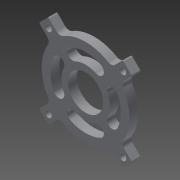
# Autodesk Inventor part: Colossus_7kW_Stator
Saved by Autodesk Inventor 2016 (Build 200138000, 138)
## iProperties
Created: 2014-11-23
Part Number: Colossus_7kW_Stator
Material: Générique
Document SubType Name: Modeling
Designer: Yann
Density: 1 g/cm^3
Appearance: Par défaut
Author: Yann
Autodesk Inventor part; units mm, degrees
ref_plane "YZ Plane" through (0, 0, 0) normal (1, 0, 0) x (0, 1, 0)
ref_plane "XZ Plane" through (0, 0, 0) normal (0, 1, 0) x (-1, 0, 0)
ref_plane "XY Plane" through (0, 0, 0) normal (0, 0, 1) x (1, 0, 0)
sketch "Esquisse1" plane through (0, 0, 0) normal (0, 1, 0) x (-1, 0, 0)
  circle A0 centre (33.9411, 33.9411) radius 3
  line L0 (0, -58.8171) -> (0, 58.8171) projected
  line L1 (-58.8171, 0) -> (58.8171, 0) projected
  line L2 (0, 0) -> (33.9411, 33.9411) construction
  line L3 (26.6119, 35.0971) -> (33.234, 41.7193)
  line L4 (34.6482, 41.7193) -> (41.7193, 34.6482)
  line L5 (41.7193, 33.234) -> (35.0971, 26.6119)
  arc A1 (34.6482, 41.7193) -> (33.234, 41.7193) centre (33.9411, 41.0122) ccw
  arc A2 (41.7193, 33.234) -> (41.7193, 34.6482) centre (41.0122, 33.9411) ccw
  arc A3 (11.636, 24.364) -> (-11.636, 24.364) centre (0, 0) ccw construction
  arc A4 (13.7909, 28.8758) -> (-13.7909, 28.8758) centre (0, 0) ccw
  arc A5 (9.4812, 19.8521) -> (-9.4812, 19.8521) centre (0, 0) ccw
  arc A6 (9.4812, 19.8521) -> (13.7909, 28.8758) centre (11.636, 24.364) ccw
  arc A7 (-13.7909, 28.8758) -> (-9.4812, 19.8521) centre (-11.636, 24.364) ccw
  circle A8 centre (0, 0) radius 16
  arc A9 (20.5123, 34.3402) -> (0, 40) centre (0, 0) ccw
  arc A10 (40, 0) -> (34.3402, 20.5123) centre (0, 0) ccw
  arc A11 (20.5123, 34.3402) -> (26.6119, 35.0971) centre (23.0763, 38.6327) ccw
  arc A12 (35.0971, 26.6119) -> (34.3402, 20.5123) centre (38.6327, 23.0763) ccw
  circle A13 centre (-33.9411, 33.9411) radius 3
  line L6 (0, 0) -> (-33.9411, 33.9411) construction
  line L7 (-35.0971, 26.6119) -> (-41.7193, 33.234)
  line L8 (-41.7193, 34.6482) -> (-34.6482, 41.7193)
  line L9 (-33.234, 41.7193) -> (-26.6119, 35.0971)
  arc A14 (-41.7193, 34.6482) -> (-41.7193, 33.234) centre (-41.0122, 33.9411) ccw
  arc A15 (-33.234, 41.7193) -> (-34.6482, 41.7193) centre (-33.9411, 41.0122) ccw
  arc A16 (-24.364, 11.636) -> (-24.364, -11.636) centre (0, 0) ccw construction
  arc A17 (-28.8758, 13.7909) -> (-28.8758, -13.7909) centre (0, 0) ccw
  arc A18 (-19.8521, 9.4812) -> (-19.8521, -9.4812) centre (0, 0) ccw
  arc A19 (-19.8521, 9.4812) -> (-28.8758, 13.7909) centre (-24.364, 11.636) ccw
  arc A20 (-28.8758, -13.7909) -> (-19.8521, -9.4812) centre (-24.364, -11.636) ccw
  arc A21 (-34.3402, 20.5123) -> (-40, 0) centre (0, 0) ccw
  arc A22 (0, 40) -> (-20.5123, 34.3402) centre (0, 0) ccw
  arc A23 (-34.3402, 20.5123) -> (-35.0971, 26.6119) centre (-38.6327, 23.0763) ccw
  arc A24 (-26.6119, 35.0971) -> (-20.5123, 34.3402) centre (-23.0763, 38.6327) ccw
  circle A25 centre (-33.9411, -33.9411) radius 3
  line L10 (0, 0) -> (-33.9411, -33.9411) construction
  line L11 (-26.6119, -35.0971) -> (-33.234, -41.7193)
  line L12 (-34.6482, -41.7193) -> (-41.7193, -34.6482)
  line L13 (-41.7193, -33.234) -> (-35.0971, -26.6119)
  arc A26 (-34.6482, -41.7193) -> (-33.234, -41.7193) centre (-33.9411, -41.0122) ccw
  arc A27 (-41.7193, -33.234) -> (-41.7193, -34.6482) centre (-41.0122, -33.9411) ccw
  arc A28 (-11.636, -24.364) -> (11.636, -24.364) centre (0, 0) ccw construction
  arc A29 (-13.7909, -28.8758) -> (13.7909, -28.8758) centre (0, 0) ccw
  arc A30 (-9.4812, -19.8521) -> (9.4812, -19.8521) centre (0, 0) ccw
  arc A31 (-9.4812, -19.8521) -> (-13.7909, -28.8758) centre (-11.636, -24.364) ccw
  arc A32 (13.7909, -28.8758) -> (9.4812, -19.8521) centre (11.636, -24.364) ccw
  arc A33 (-20.5123, -34.3402) -> (0, -40) centre (0, 0) ccw
  arc A34 (-40, 0) -> (-34.3402, -20.5123) centre (0, 0) ccw
  arc A35 (-20.5123, -34.3402) -> (-26.6119, -35.0971) centre (-23.0763, -38.6327) ccw
  arc A36 (-35.0971, -26.6119) -> (-34.3402, -20.5123) centre (-38.6327, -23.0763) ccw
  circle A37 centre (33.9411, -33.9411) radius 3
  line L14 (0, 0) -> (33.9411, -33.9411) construction
  line L15 (35.0971, -26.6119) -> (41.7193, -33.234)
  line L16 (41.7193, -34.6482) -> (34.6482, -41.7193)
  line L17 (33.234, -41.7193) -> (26.6119, -35.0971)
  arc A38 (41.7193, -34.6482) -> (41.7193, -33.234) centre (41.0122, -33.9411) ccw
  arc A39 (33.234, -41.7193) -> (34.6482, -41.7193) centre (33.9411, -41.0122) ccw
  arc A40 (24.364, -11.636) -> (24.364, 11.636) centre (0, 0) ccw construction
  arc A41 (28.8758, -13.7909) -> (28.8758, 13.7909) centre (0, 0) ccw
  arc A42 (19.8521, -9.4812) -> (19.8521, 9.4812) centre (0, 0) ccw
  arc A43 (19.8521, -9.4812) -> (28.8758, -13.7909) centre (24.364, -11.636) ccw
  arc A44 (28.8758, 13.7909) -> (19.8521, 9.4812) centre (24.364, 11.636) ccw
  arc A45 (34.3402, -20.5123) -> (40, 0) centre (0, 0) ccw
  arc A46 (0, -40) -> (20.5123, -34.3402) centre (0, 0) ccw
  arc A47 (34.3402, -20.5123) -> (35.0971, -26.6119) centre (38.6327, -23.0763) ccw
  arc A48 (26.6119, -35.0971) -> (20.5123, -34.3402) centre (23.0763, -38.6327) ccw
  circle A49 centre (0, 0) radius 16 construction
  point P0 (23.7216, 32.2069)
  point P1 (32.2069, 23.7216)
  point P2 (-32.2069, 23.7216)
  point P3 (-23.7216, 32.2069)
  point P4 (-23.7216, -32.2069)
  point P5 (-32.2069, -23.7216)
  point P6 (32.2069, -23.7216)
  point P7 (23.7216, -32.2069)
  dimension "d1" = 6
  dimension "d2" = 48
  dimension "d3" = 6
  dimension "d4" = 6
  dimension "d5" = 45
  dimension "d6" = 1
  dimension "d9" = 10
  dimension "d10" = 9
  dimension "d11" = 40
  dimension "d12" = 5
  dimension "d13" = 27
  constraints: 96 point on circle, 49 centre point, 32 end point, 17 coincident, 13 tangent, 8 point on line, 3 equal radius, 2 perpendicular, 1 parallel, 1 symmetric about line, 1 other
  measures "d1" diameter of A0
  measures "d2" distance of L2.start L2.end
  measures "d3" distance from line of L4 L2.end
  measures "d4" distance from line of L2.end L3
  measures "d5" angle of L1 L2
  measures "d6" radius of A1
  measures "d9" radial gap between concentric circles of A5 A4
  measures "d10" distance from line of A3.start L2
  measures "d11" radius of A9
  measures "d12" radius of A11
  measures "d13" radius of A3
extrude "Extrusion1" add sketch "Esquisse1" along normal blind 8 contours A33 A35 L11 A26 L12 A27 L13 A36 A34 L1 A17 A20 A18 A8 L0 A30 A31 A29 | L0 A29 A32 A30 A8 L1 A42 A43 A41 A45 A47 L15 A38 L16 A39 L17 A48 A46 | L1 A18 A19 A17 A21 A23 L7 A14 L8 A15 L9 A24 A22 L0 A4 A7 A5 A8 | A8 L0 A5 A6 A4 A9 A11 L3 A1 L4 A2 L5 A12 A10 L1 A41 A44 A42
equation "\"d4\" = d3"
